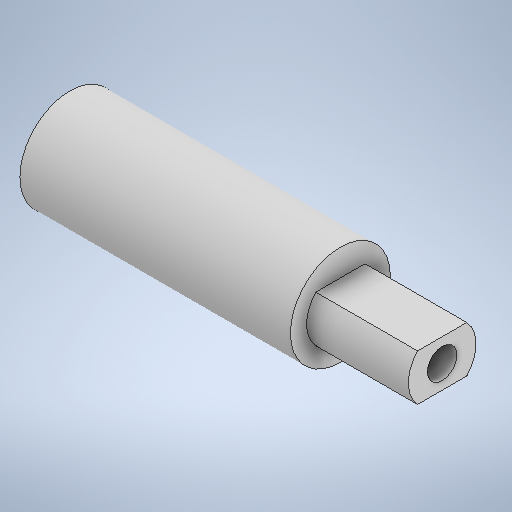
# Autodesk Inventor part: shaft shooting
Saved by Autodesk Inventor 2025.3 (Build 293356000, 356)
## iProperties
Created: 2026-04-16
Part Number: shaft shooting
Material: Generic
Document SubType Name: Modeling
Designer: lenovo
Density: 1 g/cm^3
Appearance: Default
Author: lenovo
## iProperties of the stored document shaft shooting_3DPrint.ipt
Created: 2026-04-16
Part Number: shaft shooting_3DPrint
Material: Generic
Document SubType Name: Modeling
Designer: lenovo
Density: 1 g/cm^3
Appearance: Default
Author: lenovo
Autodesk Inventor part; units mm, degrees
ref_plane "YZ Plane" through (0, 0, 0) normal (1, 0, 0) x (0, 1, 0)
ref_plane "XZ Plane" through (0, 0, 0) normal (0, 1, 0) x (-1, 0, 0)
ref_plane "XY Plane" through (0, 0, 0) normal (0, 0, 1) x (1, 0, 0)
sketch "Sketch1" plane through (0, 0, 0) normal (1, 0, 0) x (0, 1, 0)
  circle A0 centre (0, 0) radius 3.875
  dimension "d0" = 7.75
  constraints: 1 centre point, 1 coincident
  measures "d0" diameter of A0
extrude "Extrusion1" add sketch "Sketch1" along normal blind 21
sketch "Sketch2" plane through (21, 0, 0) normal (1, 0, 0) x (0, 0, -1)
  circle A0 centre (0, 0) radius 2.625
  line L0 (1.9107, -1.8) -> (-1.9107, -1.8)
  line L1 (-2.625, 0) -> (2.625, 0)
  line L2 (1.9107, 1.8) -> (-1.9107, 1.8)
  dimension "d3" = 5.25
  dimension "d4" = 1.8
  constraints: 6 end point, 4 point on circle, 2 horizontal, 2 symmetric about line, 1 centre point, 1 coincident
  measures "d3" diameter of A0
  measures "d4" distance from line of point (0, 0) L0
extrude "Extrusion2" add sketch "Sketch2" along normal blind 7.9 contours L1 A0 L2 | A0 L0 L1
sketch "Sketch3" plane through (28.9, 0, 0) normal (1, 0, 0) x (0, 0, -1)
  circle A0 centre (0, 0) radius 1.15
  dimension "d7" = 2.3
  constraints: 1 centre point, 1 coincident
  measures "d7" diameter of A0
extrude "Extrusion3" cut sketch "Sketch3" against normal through all
body "Solid1"
